Autodesk Fusion 360 part; units mm, degrees
(part 4 of 4)
  spline S180 degree 3 poles (-32.3911, -5.2354) (-32.3859, -5.2374) (-32.3746, -5.2417) (-32.356, -5.247) (-32.3351, -5.2537) (-32.311, -5.2593) (-32.2846, -5.2661) (-32.2552, -5.2726) (-32.2232, -5.2795) (-32.201, -5.2841) (-32.1895, -5.2865) knots 0 0 0 0 0.079906 0.173499 0.27898 0.3966 0.528922 0.672479 0.830442 1 1 1 1
  line L320 (-18.0888, -6.8225) -> (-18.0888, -6.6495)
  line L321 (-17.2426, -5.7841) -> (-16.9695, -5.8367)
  line L322 (-31.3051, -6.1411) -> (-31.709, -6.0641)
  spline S181 degree 3 poles (-32.1435, -4.3911) (-32.1589, -4.3908) (-32.1896, -4.3904) (-32.2352, -4.3866) (-32.2801, -4.381) (-32.324, -4.3729) (-32.3672, -4.3623) (-32.4095, -4.3494) (-32.451, -4.334) (-32.4916, -4.3167) (-32.5304, -4.297) (-32.5672, -4.2753) (-32.6019, -4.2516) (-32.634, -4.2258) (-32.6636, -4.1979) (-32.6911, -4.1684) (-32.7164, -4.1369) (-32.7387, -4.1032) (-32.7589, -4.0685) (-32.7763, -4.033) (-32.791, -3.9971) (-32.8036, -3.961) (-32.8128, -3.9242) (-32.8193, -3.8869) (-32.8239, -3.8493) (-32.8242, -3.8241) (-32.8244, -3.8114) knots 0 0 0 0 0.046399 0.092322 0.137563 0.182282 0.226624 0.271023 0.315334 0.359589 0.403501 0.446168 0.48819 0.529536 0.570022 0.610301 0.650801 0.691399 0.731746 0.771348 0.810109 0.848303 0.886216 0.924147 0.962031 1 1 1 1
  spline S182 degree 3 poles (-31.8616, -3.5572) (-31.8479, -3.5701) (-31.8208, -3.5957) (-31.7859, -3.6389) (-31.7558, -3.6846) (-31.7318, -3.7338) (-31.7126, -3.7856) (-31.6997, -3.8407) (-31.6912, -3.8985) (-31.6902, -3.9381) (-31.6898, -3.9584) knots 0 0 0 0 0.125477 0.247793 0.368802 0.48933 0.611524 0.736433 0.865114 1 1 1 1
  line L323 (-17.685, -6.8225) -> (-18.0888, -6.8225)
  line L324 (-32.8051, -5.1603) -> (-32.6068, -5.2008)
  line L325 (-31.709, -5.8911) -> (-31.4359, -5.9436)
  line L326 (-17.5119, -6.8225) -> (-17.5119, -7.2264)
  line L327 (-31.709, -6.0641) -> (-31.709, -6.2564)
  line L328 (-31.8436, -6.218) -> (-31.8436, -6.0257)
  line L329 (-17.5119, -6.2456) -> (-17.5119, -6.6495)
  line L330 (-17.685, -6.2456) -> (-17.5119, -6.2456)
  line L331 (-32.8051, -5.3364) -> (-32.8051, -5.1603)
  line L332 (-17.5119, -6.6495) -> (-17.108, -6.6495)
  spline S183 degree 3 poles (-18.343, -5.919) (-18.3475, -5.8974) (-18.3562, -5.8553) (-18.3574, -5.8123) (-18.358, -5.7913) knots 0 0 0 0 0.511633 1 1 1 1
  spline S184 degree 3 poles (-18.3027, -5.6314) (-18.2954, -5.6242) (-18.2809, -5.61) (-18.2535, -5.595) (-18.2224, -5.5861) (-18.2003, -5.5851) (-18.1889, -5.5846) knots 0 0 0 0 0.241533 0.480086 0.728963 1 1 1 1
  line L333 (-31.8436, -5.718) -> (-31.709, -5.7564)
  line L334 (-31.4359, -5.9436) -> (-31.3051, -6.1411)
  line L335 (-32.3445, -4.5897) -> (-31.709, -4.7312)
  line L336 (-31.709, -4.7312) -> (-31.709, -4.9073)
  spline S185 degree 3 poles (-32.5615, -4.7327) (-32.571, -4.7332) (-32.5893, -4.7342) (-32.6154, -4.7404) (-32.6376, -4.7528) (-32.6568, -4.7688) (-32.6716, -4.7899) (-32.6825, -4.815) (-32.6887, -4.8445) (-32.6894, -4.8655) (-32.6898, -4.8766) knots 0 0 0 0 0.130697 0.251063 0.363318 0.475137 0.590039 0.712809 0.847528 1 1 1 1
  line L337 (-18.1928, -5.9493) -> (-18.343, -5.919)
  line L338 (-19.7963, 14.32) -> (-19.7963, 13.7815)
  line L339 (-18.7184, -10.1726) -> (-18.7184, -7.6726)
  spline S186 degree 3 poles (-18.1167, -4.4451) (-18.1104, -4.4453) (-18.0968, -4.4456) (-18.0747, -4.4475) (-18.0496, -4.4506) (-18.0213, -4.4544) (-17.99, -4.4601) (-17.9555, -4.4661) (-17.9179, -4.4742) (-17.8918, -4.4798) (-17.8782, -4.4827) knots 0 0 0 0 0.078305 0.169301 0.274392 0.392282 0.523404 0.668633 0.827246 1 1 1 1
  spline S187 degree 3 poles (-18.0083, -5.7841) (-18.0178, -5.7823) (-18.0358, -5.779) (-18.0614, -5.7749) (-18.084, -5.7713) (-18.1035, -5.7683) (-18.12, -5.7659) (-18.1334, -5.764) (-18.144, -5.763) (-18.15, -5.7628) (-18.1525, -5.7627) knots 0 0 0 0 0.198784 0.376221 0.532667 0.670161 0.782601 0.87611 0.948465 1 1 1 1
  line L340 (-20.5655, 14.32) -> (-20.5655, 14.5507)
  line L341 (-20.027, 14.5507) -> (-20.027, 15.0892)
  spline S188 degree 3 poles (-18.1525, -5.7627) (-18.1579, -5.763) (-18.1682, -5.7634) (-18.1826, -5.7667) (-18.195, -5.7722) (-18.2056, -5.7801) (-18.214, -5.7911) (-18.2196, -5.8051) (-18.2228, -5.822) (-18.2232, -5.8342) (-18.2234, -5.8409) knots 0 0 0 0 0.133915 0.253294 0.361774 0.467629 0.576952 0.697757 0.836473 1 1 1 1
  line L342 (-17.2426, -5.4541) -> (-18.3388, -5.2294)
  line L343 (-19.2578, 14.5507) -> (-19.2578, 14.32)
  spline S189 degree 3 poles (-17.2234, -3.8514) (-17.2237, -3.8672) (-17.2242, -3.8983) (-17.2307, -3.9435) (-17.2395, -3.9867) (-17.2535, -4.0272) (-17.2703, -4.0657) (-17.2921, -4.1011) (-17.3166, -4.1349) (-17.3456, -4.1655) (-17.3773, -4.1937) (-17.4124, -4.2177) (-17.45, -4.2384) (-17.4903, -4.2551) (-17.5333, -4.2681) (-17.5789, -4.2773) (-17.6271, -4.2832) (-17.6602, -4.2838) (-17.6771, -4.2841) knots 0 0 0 0 0.067163 0.131444 0.193598 0.253643 0.312774 0.371272 0.429893 0.489702 0.549602 0.609458 0.669531 0.731222 0.794246 0.859725 0.928167 1 1 1 1
  line L344 (-17.2426, -5.2781) -> (-17.2426, -5.4541)
  line L345 (-18.3388, -5.0533) -> (-18.1405, -5.0939)
  line L346 (-17.2426, -4.8003) -> (-17.9563, -4.6453)
  spline S190 degree 3 poles (-17.6771, -4.2841) (-17.6926, -4.2839) (-17.7233, -4.2834) (-17.7689, -4.2796) (-17.8138, -4.274) (-17.8577, -4.2659) (-17.9008, -4.2553) (-17.9432, -4.2425) (-17.9846, -4.227) (-18.0252, -4.2098) (-18.064, -4.19) (-18.1009, -4.1683) (-18.1355, -4.1446) (-18.1677, -4.1188) (-18.1972, -4.0909) (-18.2247, -4.0614) (-18.2501, -4.0299) (-18.2724, -3.9962) (-18.2925, -3.9615) (-18.31, -3.926) (-18.3246, -3.8901) (-18.3372, -3.854) (-18.3465, -3.8172) (-18.3529, -3.7799) (-18.3575, -3.7423) (-18.3579, -3.7171) (-18.358, -3.7044) knots 0 0 0 0 0.046399 0.092322 0.137563 0.182282 0.226624 0.271023 0.315334 0.359589 0.403501 0.446168 0.48819 0.529536 0.570022 0.610301 0.650801 0.691399 0.731746 0.771348 0.810109 0.848303 0.886216 0.924147 0.962031 1 1 1 1
  line L347 (-18.7184, -7.6726) -> (-16.2184, -7.6726)
  spline S191 degree 3 poles (-17.9214, -3.2648) (-17.8955, -3.2654) (-17.8446, -3.2665) (-17.77, -3.2755) (-17.6988, -3.2898) (-17.6309, -3.3098) (-17.5666, -3.3362) (-17.5057, -3.3681) (-17.448, -3.4057) (-17.4129, -3.4353) (-17.3953, -3.4502) knots 0 0 0 0 0.136455 0.267383 0.394171 0.517765 0.638894 0.758991 0.878725 1 1 1 1
  circle A0 centre (-20.7684, -8.9226) radius 0.5
  circle A1 centre (-17.4684, -8.9226) radius 0.5
  spline S192 degree 3 poles (-18.358, -4.7117) (-18.3578, -4.7019) (-18.3573, -4.6829) (-18.3539, -4.6551) (-18.3486, -4.6286) (-18.3412, -4.6036) (-18.3311, -4.5802) (-18.319, -4.5582) (-18.305, -4.5373) (-18.2883, -4.5186) (-18.2704, -4.5015) (-18.2515, -4.4864) (-18.2314, -4.4736) (-18.2104, -4.4631) (-18.1883, -4.4549) (-18.1654, -4.4492) (-18.1414, -4.4459) (-18.1251, -4.4454) (-18.1167, -4.4451) knots 0 0 0 0 0.072499 0.141692 0.208769 0.273502 0.336062 0.398225 0.460571 0.523024 0.584826 0.64489 0.70331 0.761755 0.819879 0.878381 0.937945 1 1 1 1
  circle A2 centre (-17.4684, 13.6774) radius 0.5
  spline S193 degree 3 poles (-17.3953, -3.4502) (-17.3816, -3.4632) (-17.3544, -3.4887) (-17.3196, -3.5319) (-17.2894, -3.5776) (-17.2655, -3.6268) (-17.2462, -3.6787) (-17.2333, -3.7337) (-17.2248, -3.7915) (-17.2239, -3.8311) (-17.2234, -3.8514) knots 0 0 0 0 0.125477 0.247793 0.368802 0.48933 0.611524 0.736433 0.865114 1 1 1 1
  spline S194 degree 3 poles (-17.9247, -5.1284) (-17.9196, -5.1304) (-17.9083, -5.1347) (-17.8897, -5.14) (-17.8687, -5.1467) (-17.8447, -5.1523) (-17.8183, -5.1591) (-17.7889, -5.1656) (-17.7569, -5.1725) (-17.7346, -5.1771) (-17.7231, -5.1795) knots 0 0 0 0 0.079906 0.173499 0.27898 0.3966 0.528922 0.672479 0.830442 1 1 1 1
  spline S195 degree 3 poles (-18.0951, -4.6257) (-18.1047, -4.6262) (-18.123, -4.6272) (-18.1491, -4.6334) (-18.1712, -4.6458) (-18.1904, -4.6618) (-18.2052, -4.6829) (-18.2162, -4.708) (-18.2224, -4.7375) (-18.2231, -4.7585) (-18.2234, -4.7697) knots 0 0 0 0 0.130697 0.251063 0.363318 0.475137 0.590039 0.712809 0.847528 1 1 1 1
  line L348 (-17.2426, -4.6242) -> (-17.2426, -4.8003)
  line L349 (-20.5655, 14.5507) -> (-20.027, 14.5507)
  line L350 (-19.7963, 15.0892) -> (-19.7963, 14.5507)
  line L351 (-29.7035, 14.4482) -> (-29.4727, 14.3969)
  circle A3 centre (-31.4684, -8.9226) radius 0.5
  line L352 (-29.7035, 13.6789) -> (-29.7035, 14.4482)
  line L353 (-17.8782, -4.4827) -> (-17.2426, -4.6242)
  spline S196 degree 3 poles (-18.1405, -5.0939) (-18.1578, -5.0785) (-18.1913, -5.0489) (-18.2353, -5.0012) (-18.2732, -4.9538) (-18.3039, -4.9061) (-18.3281, -4.8578) (-18.3453, -4.8094) (-18.3562, -4.7606) (-18.3574, -4.7279) (-18.358, -4.7117) knots 0 0 0 0 0.152822 0.295762 0.428272 0.553392 0.670988 0.784111 0.892453 1 1 1 1
  line L354 (-29.4727, 14.3969) -> (-29.4727, 13.6276)
  line L355 (-20.027, 14.32) -> (-20.5655, 14.32)
  line L356 (-20.027, 15.0892) -> (-19.7963, 15.0892)
  line L357 (-17.7231, -5.1795) -> (-17.2426, -5.2781)
  circle A4 centre (-28.1684, -8.9226) radius 0.5
  line L358 (-16.2184, -10.1726) -> (-18.7184, -10.1726)
  line L359 (-20.027, 13.7815) -> (-20.027, 14.32)
  circle A5 centre (-31.4684, 13.6774) radius 0.5
  spline S197 degree 3 poles (-18.2234, -4.7697) (-18.223, -4.7823) (-18.222, -4.8076) (-18.2145, -4.8453) (-18.202, -4.8823) (-18.1852, -4.9186) (-18.1642, -4.9533) (-18.1398, -4.9859) (-18.1119, -5.0162) (-18.0806, -5.0437) (-18.0461, -5.0689) (-18.0085, -5.0912) (-17.968, -5.1117) (-17.9394, -5.1228) (-17.9247, -5.1284) knots 0 0 0 0 0.076337 0.152702 0.231094 0.31171 0.393628 0.475252 0.557411 0.641365 0.726626 0.814766 0.905349 1 1 1 1
  line L360 (-19.2578, 14.32) -> (-19.7963, 14.32)
  spline S198 degree 3 poles (-17.9563, -4.6453) (-17.9704, -4.6424) (-17.9969, -4.637) (-18.0341, -4.6305) (-18.0663, -4.6266) (-18.0861, -4.626) (-18.0951, -4.6257) knots 0 0 0 0 0.307639 0.576784 0.807205 1 1 1 1
  line L361 (-19.7963, 13.7815) -> (-20.027, 13.7815)
  line L362 (-16.2184, -7.6726) -> (-16.2184, -10.1726)
  line L363 (-19.7963, 14.5507) -> (-19.2578, 14.5507)
  spline S199 degree 3 poles (-18.358, -3.7044) (-18.3574, -3.684) (-18.3563, -3.6437) (-18.3458, -3.5847) (-18.3285, -3.5286) (-18.3049, -3.4759) (-18.2753, -3.4273) (-18.2396, -3.3844) (-18.1979, -3.348) (-18.1507, -3.318) (-18.0991, -3.2941) (-18.0433, -3.277) (-17.9836, -3.2665) (-17.9425, -3.2654) (-17.9214, -3.2648) knots 0 0 0 0 0.08805 0.173362 0.256795 0.339941 0.4214 0.500643 0.579137 0.659 0.740185 0.823206 0.909367 1 1 1 1
  line L364 (-29.4727, 13.6276) -> (-29.7035, 13.6789)
  line L365 (-18.3388, -5.2294) -> (-18.3388, -5.0533)
  line L366 (-34.1184, 15.9774) -> (-34.1184, -11.3226)
  line L367 (-34.1184, -11.3226) -> (-14.8184, -11.3226)
  line L368 (-14.8184, -11.3226) -> (-14.8184, 15.9774)
  line L369 (-41, 16.3) -> (80, 16.3)
  line L370 (-14.8184, 15.9774) -> (-14.8184, 16.3)
  line L371 (-33.1184, 15.9774) -> (-33.1184, 16.3)
  line L372 (-34.1184, 15.9774) -> (-34.1184, 16.3)
  line L373 (-34.1184, 16.3) -> (-33.1184, 16.3)
  line L374 (-15.8184, 15.9774) -> (-15.8184, 16.3)
  line L375 (-15.8184, 16.3) -> (-14.8184, 16.3)
  point P0 (-20, 10)
  dimension "d143" = 1
  constraint vertical L370
  constraint vertical L371
  constraint vertical L372
  constraint horizontal L373
  constraint vertical L374
  constraint horizontal L375
extrude "Extruir33" add sketch "Boceto35" along normal blind 2 contours L11 L29 L46 L47 L179 L190 L210 L366 L367 L368 L369 L370 L371 L372 L373 L374 L375 | A1 | A2 | A3 | A5 bodies 1
sketch "Boceto36" plane through (0, 0, 19.3) normal (0, 0, 1) x (1, 0, 0)
  line L0 (33.1184, 0) -> (15.8184, 0)
  line L1 (15.8184, 0) -> (24.4684, 0)
  line L2 (33.1184, 0) -> (24.4684, 0)
  line L3 (24.4684, 0) -> (24.4684, 4)
  line L4 (24.4684, 4) -> (28.4684, 4)
  line L5 (24.4684, 4) -> (20.4684, 4)
  line L6 (20.4684, 4) -> (20.4684, 2)
  circle A0 centre (20.4684, 2) radius 2
  line L7 (28.4684, 4) -> (28.4684, 2)
  circle A1 centre (28.4684, 2) radius 2
  dimension "d146" = 4
  dimension "d147" = 4
  dimension "d148" = 4
  dimension "d149" = 2
  dimension "d150" = 4
  dimension "d151" = 2
  dimension "d152" = 4
  constraint coincident L0.end L1.start
  constraint midpoint L0 L1.end
  constraint coincident L0.start L2.start
  constraint perpendicular L0 L3
  constraint perpendicular L3 L4
  constraint perpendicular L3 L5
  constraint perpendicular L5 L6
  constraint coincident L6.end A0.centre
  constraint perpendicular L4 L7
  constraint coincident L7.end A1.centre
  measures "d146" distance of L1.end L3.end
  measures "d147" distance of L3.end L4.end
  measures "d148" distance of L3.end L5.end
  measures "d149" distance of L5.end L6.end
  measures "d150" diameter of A0
  measures "d151" distance of L4.end L7.end
  measures "d152" diameter of A1
extrude "Extruir34" cut sketch "Boceto36" against normal blind 10 bodies 1
extrude "Extruir2" [rolled back] along distance -0.5 taper angle 0
